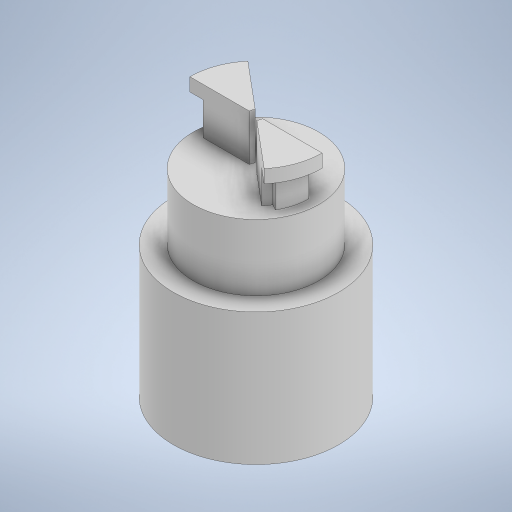
# Autodesk Inventor part: kumi3
Saved by Autodesk Inventor 2023.2 (Build 272271000, 271)
## iProperties
Created: 2022-12-16
Part Number: kumi3
Material: 一般
Document SubType Name: Modeling
Designer: 千葉 俊輔
Density: 1 g/cm^3
Appearance: 既定
Author: 千葉 俊輔
Autodesk Inventor part; units mm, degrees
ref_plane "YZ Plane" through (0, 0, 0) normal (1, 0, 0) x (0, 1, 0)
ref_plane "XZ Plane" through (0, 0, 0) normal (0, 1, 0) x (-1, 0, 0)
ref_plane "XY Plane" through (0, 0, 0) normal (0, 0, 1) x (1, 0, 0)
sketch "スケッチ1" plane through (0, 0, 0) normal (0, 1, 0) x (-1, 0, 0)
  circle A0 centre (0, 0) radius 12.5
  dimension "d0" = 25
  constraints: 1 centre point, 1 coincident
  measures "d0" diameter of A0
extrude "押し出し1" add sketch "スケッチ1" along normal blind 20
sketch "スケッチ2" plane through (0, 20, 0) normal (0, 1, 0) x (1, 0, 0)
  circle A0 centre (0, 0) radius 9.5
  dimension "d3" = 19
  constraints: 1 centre point, 1 coincident
  measures "d3" diameter of A0
extrude "押し出し2" add sketch "スケッチ2" along normal blind 10
sketch "スケッチ3" plane through (0, 30, 0) normal (0, 1, 0) x (1, 0, 0)
  arc A0 (-6.9282, 4) -> (-8, 0) centre (0, 0) ccw
  line L0 (0, 0) -> (-6.9282, 4) construction
  line L1 (0, 0) -> (-8, 0) construction
  circle A1 centre (0, 0) radius 9.5 projected
  arc A2 (-5.3623, 4.4995) -> (-6.0622, 3.5) centre (0, 0) ccw
  line L2 (0, 0) -> (-5.3623, 4.4995) construction
  line L3 (0, 0) -> (-6.0622, 3.5) construction
  arc A3 (6.9282, -4) -> (8, 0) centre (0, 0) ccw
  line L4 (0, 0) -> (6.9282, -4) construction
  line L5 (0, 0) -> (8, 0) construction
  arc A4 (5.3623, -4.4995) -> (6.0622, -3.5) centre (0, 0) ccw
  line L6 (0, 0) -> (5.3623, -4.4995) construction
  line L7 (0, 0) -> (6.0622, -3.5) construction
  line L8 (-5.3623, 4.4995) -> (0, 0)
  line L9 (-6.9282, 4) -> (0, 0)
  line L10 (-8, 0) -> (0, 0)
  line L11 (0, 0) -> (8, 0)
  line L12 (0, 0) -> (6.9282, -4)
  line L13 (0, 0) -> (5.3623, -4.4995)
  point P0 (-6.0622, 3.5)
  point P1 (6.0622, -3.5)
  dimension "d6" = 8
  dimension "d7" = 30
  dimension "d8" = 7
  dimension "d9" = 10
  dimension "d10" = 8
  dimension "d11" = 30
  dimension "d12" = 7
  dimension "d13" = 10
  constraints: 28 end point, 8 point on circle, 5 collinear, 4 centre point, 4 coincident, 1 horizontal, 1 point on line
  measures "d6" radius of A0
  measures "d7" angle of L0 L1
  measures "d8" radius of A2
  measures "d9" angle of L2 L3
  measures "d10" radius of A3
  measures "d11" angle of L4 L5
  measures "d12" radius of A4
  measures "d13" angle of L6 L7
extrude "押し出し3" add sketch "スケッチ3" along normal blind 5 contours L9 L10 A0 | L11 A3 L12 | L12 A4 L13 | A2 L8 L9
sketch "スケッチ4" plane through (0, 35, 0) normal (0, 1, 0) x (1, 0, 0)
  line L0 (8, 0) -> (0, 0) projected
  arc A0 (-7.6604, 6.4279) -> (-10, 0) centre (0, 0) ccw
  line L1 (0, 0) -> (-7.6604, 6.4279) construction
  line L2 (0, 0) -> (-10, 0) construction
  line L3 (0, 0) -> (5.3623, -4.4995) projected
  arc A1 (7.6604, -6.4279) -> (10, 0) centre (0, 0) ccw
  line L4 (0, 0) -> (7.6604, -6.4279) construction
  line L5 (0, 0) -> (10, 0) construction
  line L6 (-7.6604, 6.4279) -> (0, 0)
  line L7 (0, 0) -> (-10, 0)
  line L8 (0, 0) -> (-10, 0)
  line L9 (0, 0) -> (10, 0)
  line L10 (-8, 0) -> (0, 0) projected
  line L11 (0, 0) -> (7.6604, -6.4279)
  dimension "d16" = 10
  dimension "d17" = 40
  dimension "d18" = 10
  dimension "d19" = 40
  constraints: 18 end point, 4 point on circle, 2 centre point, 2 coincident, 2 collinear, 1 horizontal
  measures "d16" radius of A0
  measures "d17" angle of L1 L2
  measures "d18" radius of A1
  measures "d19" angle of L4 L5
extrude "押し出し4" add sketch "スケッチ4" along normal blind 2
sketch "スケッチ5" plane through (0, 37, 0) normal (0, 1, 0) x (1, 0, 0)
  line L0 (0, 0) -> (-8, 0) projected
  circle A0 centre (0, 0) radius 1
  dimension "d22" = 2
  constraints: 1 centre point, 1 coincident
  measures "d22" diameter of A0
extrude "押し出し5" cut sketch "スケッチ5" against normal blind 7
